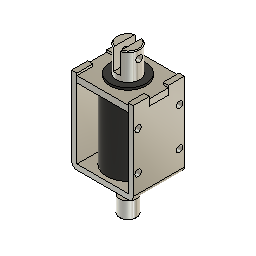
413 Large Solenoid (Autodesk Fusion 360 design; units mm, degrees)
Autodesk Fusion 360 part; units mm, degrees
sketch "profile case" plane through (0, 0, 0) normal (0, 1, 0) x (1, 0, 0)
  line L0 (-14.5, -39.5) -> (14.5, -39.5)
  line L1 (14.5, -39.5) -> (14.5, 0)
  line L2 (14.5, 0) -> (-14.5, 0)
  line L3 (-14.5, 0) -> (-14.5, -39.5)
  line L4 (-12, -39.5) -> (-12, -2.5)
  line L5 (-12, -2.5) -> (12, -2.5)
  line L6 (12, -2.5) -> (12, -39.5)
  line L7 (-12, -38.5) -> (12, -38.5)
  line L8 (-12, -35.5) -> (12, -35.5)
  dimension "d1" = 39.5
  dimension "d2" = 29
  dimension "d3" = 2.5
  dimension "d4" = 2.5
  dimension "d5" = 2.5
  dimension "d6" = 1
  dimension "d7" = -3
  constraint horizontal L0
  constraint vertical L1
  constraint horizontal L2
  constraint vertical L3
  constraint midpoint origin L2
  constraint coincident L0 L4.start
  constraint perpendicular L0 L4
  constraint perpendicular L4 L5
  constraint perpendicular L0 L6
  constraint coincident L0 L6.end
  constraint coincident L4 L7.start
  constraint coincident L6 L7.end
  constraint perpendicular L6 L7
  measures "d1" distance of L0.end L1.end
  measures "d2" distance of L0.start L0.end
  measures "d3" distance of L1 L6
  measures "d4" distance of L3 L4
  measures "d5" distance of L2 L5
  measures "d6" distance of L0 L7
extrude "Extrude1" add sketch "profile case" along normal blind 24 contours L0 L1 L2 L3 L4 L5 L6 makes body 1
extrude "Extrude2" add sketch "profile case" along normal blind 24 separate body contours L4 L6 L7 L8 makes body 2
fillet "Fillet1" radius 2.5 2 edges at (-14.5, 12, 0) (14.5, 12, 0) on bodies 1
sketch "top cover" plane through (0, 0, 0) normal (1, 0, 0) x (0, 1, 0)
  line L0 (0, 39.5) -> (24, 39.5)
  line L1 (0, 39.5) -> (0, 35.5)
  line L2 (0, 35.5) -> (24, 35.5)
  line L3 (24, 35.5) -> (24, 39.5)
  line L4 (12, 39.5) -> (12, 35.5) construction
  line L5 (16.5, 39.5) -> (16.5, 35.5)
  line L6 (7.5, 39.5) -> (7.5, 35.5)
  line L7 (0, 38.5) -> (24, 38.5)
  dimension "d13" = 4
  dimension "d14" = 4.5
  dimension "d17" = 1
  constraint coincident L0.start L1.start
  constraint perpendicular L0 L1
  constraint perpendicular L1 L2
  constraint coincident L0.end L3.end
  constraint perpendicular L0 L3
  constraint midpoint L0 L4.start
  constraint midpoint L2 L4.end
  constraint coincident L0 L5.start
  constraint coincident L2 L5.end
  constraint perpendicular L2 L5
  constraint symmetric L4 L5.start L6.start
  constraint symmetric L4 L5.end L6.end
  constraint coincident L1 L7.start
  constraint coincident L3 L7.end
  constraint perpendicular L3 L7
  measures "d13" distance of L2.end L0.end
  measures "d14" distance of L4 L5
  measures "d17" distance of L0 L7
extrude "Extrude3" cut sketch "top cover" along normal mid plane 38 contours L0 L5 L6 L7 | L2 L5 L6 L7 bodies 1
extrude "Extrude4" add sketch "top cover" along normal blind 2.5 from surface at 12 contours L2 L5 L6 L7 bodies 2
mirror "Mirror1" about plane through (0, 0, 0) normal (1, 0, 0) of "Extrude4"
sketch "piston" plane through (0, 0, 0) normal (0, 0, 1) x (1, 0, 0)
  circle A0 centre (0, 12) radius 1.75
  circle A1 centre (0, 12) radius 4
  line L0 (0, 12) -> (0, 0) construction
  circle A2 centre (0, 12) radius 1.55
  circle A3 centre (0, 12) radius 10
  dimension "d22" = 3.5
  dimension "d23" = 8
  dimension "d24" = 12
  dimension "d27" = 0.2
  dimension "d36" = 20
  constraint concentric A0 A1
  constraint coincident A0.centre A1.centre
  constraint coincident L0.end origin
  constraint vertical L0
  constraint concentric A0 A2
  constraint concentric A0 A3
  measures "d22" diameter of A0
  measures "d23" diameter of A1
  measures "d24" distance of A0.centre L0.end
  measures "d27" distance of A0 A2
  measures "d36" diameter of A3
extrude "Extrude5" cut sketch "piston" along normal up to surface (2.5 mm away) contours A0 | A2 bodies 1
extrude "Extrude6" add sketch "piston" against normal blind 9.7 separate body contours A2 makes body 3
extrude "Extrude7" add sketch "piston" along normal blind 2.5 contours A2 bodies 3
extrude "Extrude8" add sketch "piston" against normal blind 8 from surface at -9.7 contours A0 | A1 | A2 bodies 3
chamfer "Chamfer1" distance 0.4 angle 45 1 edges at (-3.7293, 13.4465, -17.7) on bodies 3
extrude "Extrude9" add sketch "piston" along normal blind 33.5 from surface at 2.5 separate body contours A0 | A1 | A2 | A3 makes body 4
sketch "holes" plane through (0, 0, 0) normal (1, 0, 0) x (0, 1, 0)
  circle A0 centre (2.25, 29) radius 1.5
  line L0 (2.25, 29) -> (21.75, 29) construction
  circle A1 centre (21.75, 29) radius 1.5
  circle A2 centre (21.75, 11) radius 1.5
  circle A3 centre (2.25, 11) radius 1.5
  line L1 (2.25, 11) -> (2.25, 29) construction
  line L2 (21.75, 11) -> (2.25, 11) construction
  line L3 (21.75, 11) -> (21.75, 29) construction
  line L4 (12, 11) -> (12, 0) construction
  line L5 (12, 0) -> (0, 0) construction
  dimension "d40" = 3
  dimension "d41" = 3
  dimension "d42" = 3
  dimension "d43" = 3
  dimension "d44" = 18
  dimension "d45" = 29
  dimension "d46" = 19.5
  dimension "d47" = 12
  constraint coincident A0.centre L0.start
  constraint horizontal L0
  constraint coincident L0.end A1.centre
  constraint coincident A3.centre L1.start
  constraint coincident A2.centre L2.start
  constraint perpendicular L0 L3
  constraint perpendicular L0 L1
  constraint perpendicular L1 L2
  constraint midpoint L2 L4.start
  constraint perpendicular L2 L4
  constraint coincident L5.end origin
  constraint perpendicular L4 L5
  measures "d40" diameter of A0
  measures "d41" diameter of A1
  measures "d42" diameter of A2
  measures "d43" diameter of A3
  measures "d44" distance of A2.centre L0.end
  measures "d45" distance of L5.end L0
  measures "d46" distance of A0.centre L0.end
  measures "d47" distance of L4.end L5.end
extrude "Extrude10" cut sketch "holes" along normal blind 16 bodies 1
sketch "top piston" plane through (0, 0, 0) normal (0, 0, 1) x (1, 0, 0)
  circle A0 centre (0, 12) radius 5.4
  line L0 (1.6, 6) -> (-1.6, 6)
  line L1 (-1.6, 6) -> (-1.6, 18)
  line L2 (-1.6, 18) -> (1.6, 18)
  line L3 (1.6, 18) -> (1.6, 6)
  line L4 (1.6, 12) -> (0, 12) construction
  line L5 (0, 18) -> (0, 12) construction
  line L6 (0, 12) -> (0, 0) construction
  circle A1 centre (0, 12) radius 8.45
  dimension "d50" = 10.8
  dimension "d51" = 3.2
  dimension "d52" = 12
  dimension "d53" = 12
  dimension "d60" = 16.9
  constraint horizontal L0
  constraint vertical L1
  constraint horizontal L2
  constraint vertical L3
  constraint midpoint L3 L4.start
  constraint coincident A0.centre L4.end
  constraint horizontal L4
  constraint midpoint L2 L5.start
  constraint perpendicular L4 L5
  constraint coincident L6.end origin
  constraint vertical L6
  measures "d50" diameter of A0
  measures "d51" distance of L1.end L2.end
  measures "d52" distance of L0.end L1.end
  measures "d53" distance of A0.centre L6.end
  measures "d60" diameter of A1
extrude "Extrude11" add sketch "top piston" along normal blind 13.5 from surface at 38.5 separate body contours A0 L3 | A0 L1 L3 | A0 L1 makes body 5
sketch "top hole" plane through (0, 0, 0) normal (1, 0, 0) x (0, 1, 0)
  circle A0 centre (12, 48) radius 1.5
  line L0 (12, 48) -> (12, 0) construction
  line L1 (12, 0) -> (0, 0) construction
  line L2 (17.4, 52) -> (6.6, 52)
  dimension "d65" = 3
  dimension "d66" = 12
  dimension "d68" = 4
  constraint coincident A0.centre L0.start
  constraint vertical L0
  constraint coincident L1.end origin
  constraint perpendicular L0 L1
  measures "d65" diameter of A0
  measures "d66" distance of L0.end L1.end
  measures "d68" distance of A0.centre L2
extrude "Extrude14" cut sketch "top hole" along normal mid plane 18 bodies 5
chamfer "Chamfer2" distance 0.4 angle 45 1 edges at (-5.0346, 10.0473, 52) on bodies 5
extrude "Extrude12" cut sketch "top piston" against normal blind 10 from surface at 52 contours A0 L1 L3 bodies 5
extrude "Extrude13" add sketch "top piston" along normal blind 1 from surface at 38.5 separate body contours A0 L1 L2 L3 | A0 L0 L1 L3 | A1 makes body 6
extrude "Extrude15" add sketch "top piston" along normal up to surface (36 mm away) from surface at 2.5 contours A0 L3 | A0 L1 L3 | A0 L1 bodies 3 5
extrude "Extrude16" cut sketch "top piston" along normal blind 15 from surface at 35.5 contours A0 L3 | A0 L1 L3 | A0 L1 bodies 2
move_face "OffsetFaces1" offset -0.2 1 faces at (5.3732, 12.5377, 37.5) on bodies 2
copy_body "Body->Comp1" bodies 1 removing the originals makes body 7 in component "case"
copy_body "CutPasteBodies1" bodies 2 removing the originals makes body 8 in component "case"
copy_body "CutPasteBodies2" bodies 4 removing the originals makes body 9 in component "case"
copy_body "Body->Comp2" bodies 3 removing the originals makes body 10 in component "piston"
copy_body "CutPasteBodies1'" bodies 6 removing the originals makes body 11 in component "piston"
component "case" placed x (1, 0, 0) y (0, 1, 0) z (0, 0, 1) at (0, 0, 0)
component "piston" placed x (1, 0, 0) y (0, 1, 0) z (0, 0, 1) at (0, 0, 0)
named bodies: "case", "top cover", "piston", "cylindar", "washer", "top noid"
